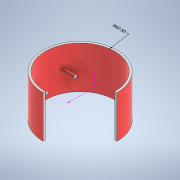
# Autodesk Inventor part: airframe
Saved by Autodesk Inventor 2022 (Build 260153000, 153)
## iProperties
Created: 2021-07-21
Part Number: airframe
Material: Generic
Document SubType Name: Modeling
Designer: WASHINGTON
Density: 1 g/cm^3
Appearance: Default
Author: WASHINGTON
Autodesk Inventor part; units mm, degrees
ref_plane "YZ Plane" through (0, 0, 0) normal (1, 0, 0) x (0, 1, 0)
ref_plane "XZ Plane" through (0, 0, 0) normal (0, 1, 0) x (-1, 0, 0)
ref_plane "XY Plane" through (0, 0, 0) normal (0, 0, 1) x (1, 0, 0)
sketch "Sketch1" plane through (0, 0, 0) normal (0, 1, 0) x (-1, 0, 0)
  arc A0 (-87.5, 0) -> (0, 87.5) centre (0, 0) ccw
  arc A1 (-82.5, 0) -> (0, 82.5) centre (0, 0) ccw
  line L0 (0, 87.5) -> (0, 82.5)
  line L1 (-82.5, 0) -> (-87.5, 0)
  dimension "d0" = 165
  dimension "d1" = 175
  dimension "d7" = 0
  dimension "d8" = 0
  constraints: 4 end point, 4 point on circle, 2 centre point, 2 coincident, 1 perpendicular, 1 vertical
  measures "d0" diameter of A1
  measures "d1" diameter of A0
  measures "d7" distance from line of point (0, 0) L0
  measures "d8" distance from line of point (0, 0) L1
extrude "Extrusion1" add sketch "Sketch1" along normal mid plane 100
sketch "Sketch3" plane through (0, 0, 0) normal (1, 0, 0) x (0, 1, 0)
  circle A0 centre (0, 34) radius 3.5
  circle A1 centre (0, -34) radius 3.5
  circle A2 centre (0, 34) radius 3.5
  circle A3 centre (0, -34) radius 3.5
  point P0 (0, 0)
  dimension "d9" = 7
  dimension "d10" = 7
  dimension "d11" = 68
  dimension "d12" = 34
  dimension "d13" = 34
  constraints: 4 centre point, 2 coincident, 2 concentric
  measures "d9" diameter of A0
  measures "d10" diameter of A1
  measures "d11" distance of A1.centre A0.centre
  measures "d12" distance of point (0, 0) A0.centre
  measures "d13" distance of point (0, 0) A1.centre
extrude "Extrusion2" add sketch "Sketch3" against normal up to next
sketch "Sketch4" plane through (0, 0, 34) normal (1, 0, 0) x (0, 0, -1)
  circle A0 centre (0, 0) radius 3.5
  circle A1 centre (68, 0) radius 3.5 projected
  circle A2 centre (68, 0) radius 3.5
  point P0 (34, 0)
  constraints: 2 centre point, 1 coincident
extrude "Extrusion3" cut sketch "Sketch4" against normal blind 45
body "Solid1"
